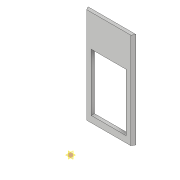
# Autodesk Inventor part: side_w_door
Saved by Autodesk Inventor 2017 (Build 210142000, 142)
## iProperties
Created: 2018-11-28
Part Number: side_w_door
Material: Generic
Document SubType Name: Modeling
Designer: jpb34
Density: 1 g/cm^3
Appearance: Default
Author: jpb34
Autodesk Inventor part; units mm, degrees
sketch "Sketch1" plane through (0, 0, 0) normal (0, 1, 0) x (-1, 0, 0)
  line L0 (95.25, -164.9778) -> (-95.25, -164.9778)
  line L1 (87.9177, -152.2778) -> (-87.9177, -152.2778)
  line L2 (95.25, -164.9778) -> (87.9177, -152.2778)
  line L3 (-95.25, -164.9778) -> (-87.9177, -152.2778)
  point P0 (0, 0)
  point P1 (0, 0)
  point P2 (0, 0)
  dimension "d0" = 190.5
  dimension "d1" = 12.7
  dimension "d3" = 120
  dimension "d4" = 0
  constraints: 8 end point, 2 coincident, 1 horizontal, 4 other
  measures "d0" distance of L0.start L0.end
  measures "d1" distance between parallel lines of L1 L0
  measures "d3" angle of L2 L1
  measures "d4" distance from line of point (0, 0) L2
extrude "Extrusion1" add sketch "Sketch1" along normal blind 381
sketch "Sketch2" plane through (95.25, 0, -164.9778) normal (0, 0, -1) x (-1, 0, 0)
  line L0 (25.4, 254) -> (165.1, 254)
  line L1 (165.1, 254) -> (165.1, 25.4)
  line L2 (165.1, 25.4) -> (25.4, 25.4)
  line L3 (25.4, 25.4) -> (25.4, 254)
  line L4 (0, 0) -> (0, 381) projected
  point P0 (95.25, 0)
  dimension "d7" = 139.7
  dimension "d8" = 25.4
  dimension "d9" = 25.4
  dimension "d10" = 228.6
  constraints: 8 end point, 2 parallel, 1 horizontal, 1 perpendicular
  measures "d7" distance of L0.start L0.end
  measures "d8" distance between parallel lines of L4 L3
  measures "d9" distance from line of L2 L4.start
  measures "d10" distance of L0.end L1.end
extrude "Extrusion2" cut sketch "Sketch2" against normal up to next
body "Solid1"
